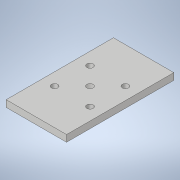
# Autodesk Inventor part: Platform A
Saved by Autodesk Inventor 2022 (Build 260153000, 153)
## iProperties
Created: 2021-01-07
Part Number: Platform A
Material: Generic
Document SubType Name: Modeling
Designer: caleb
Density: 1 g/cm^3
Appearance: Default
Author: caleb
Autodesk Inventor part; units mm, degrees
ref_plane "YZ Plane" through (0, 0, 0) normal (1, 0, 0) x (0, 1, 0)
ref_plane "XZ Plane" through (0, 0, 0) normal (0, 1, 0) x (-1, 0, 0)
ref_plane "XY Plane" through (0, 0, 0) normal (0, 0, 1) x (1, 0, 0)
sketch "Sketch1" plane through (0, 0, 0) normal (0, 1, 0) x (-1, 0, 0)
  line L0 (-14.351, 25.5) -> (14.351, 25.5)
  line L1 (14.351, 25.5) -> (14.351, -25.5)
  line L2 (14.351, -25.5) -> (-14.351, -25.5)
  line L3 (-14.351, -25.5) -> (-14.351, 25.5)
  line L4 (-14.351, 25.5) -> (14.351, -25.5) construction
  line L5 (14.351, 25.5) -> (-14.351, -25.5) construction
  point P0 (0, 0)
  dimension "d0" = 51
  dimension "d1" = 28.702
  constraints: 12 end point, 2 midpoint, 2 parallel, 1 horizontal, 1 perpendicular
  measures "d0" distance of L0.end L1.end
  measures "d1" distance of L0.start L0.end
extrude "Extrusion1" add sketch "Sketch1" along normal blind 3.175
sketch "Sketch2" plane through (0, 3.175, 0) normal (0, 1, 0) x (1, 0, 0)
  circle A0 centre (-8.4201, -8.4201) radius 1.4986
  line L0 (-14.351, 25.5) -> (-14.351, -25.5) projected
  line L1 (-14.351, -25.5) -> (14.351, -25.5) projected
  circle A1 centre (-8.4201, 8.4201) radius 1.4986
  circle A2 centre (8.4201, -8.4201) radius 1.4986
  circle A3 centre (8.4201, 8.4201) radius 1.4986
  point P0 (0, 0)
  dimension "d4" = 2.9972
  dimension "d5" = 8.4201
  dimension "d8" = 16.8402
  dimension "d11" = 16.8402
  dimension "d14" = 8.4201
  constraints: 4 centre point, 1 horizontal, 1 vertical, 6 other
  measures "d4" diameter of A0
  measures "d5" horizontal distance of A0.centre point (0, 0)
  measures "d8" distance of A0.centre A1.centre
  measures "d11" distance of A0.centre A2.centre
  measures "d14" horizontal distance of point (0, 0) A0.centre
hole "Hole1" at (8.4201, 3.175, -8.4201) at (-8.4201, 3.175, -8.4201) at (-8.4201, 3.175, 8.4201) at (8.4201, 3.175, 8.4201) direction (0, -1, 0) diameter 2.9972 end through all
sketch "Sketch3" plane through (0, 3.175, 0) normal (0, 1, 0) x (1, 0, 0)
  circle A0 centre (0, 0) radius 1.4986
  dimension "d22" = 2.9972
  constraints: 1 centre point, 1 coincident
  measures "d22" diameter of A0
extrude "Extrusion2" cut sketch "Sketch3" against normal through all
body "Solid1"
